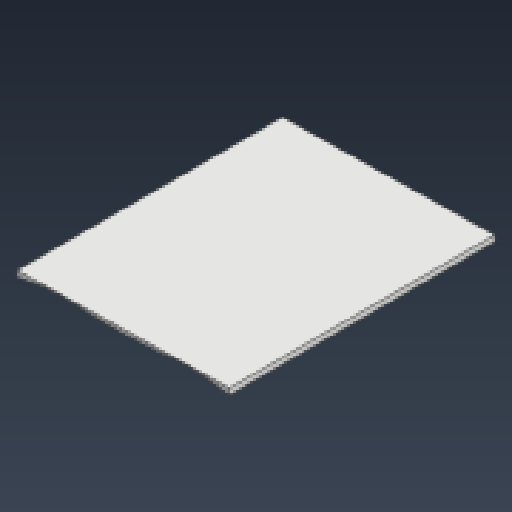
# Autodesk Inventor part: deseczka_dol_check - 6
Saved by Autodesk Inventor 2023 (Build 270158000, 158)
## iProperties
Created: 2025-12-25
Part Number: deseczka_dol_check - 6
Material: Generic
Document SubType Name: Modeling
Designer: szymo
Density: 1 g/cm^3
Appearance: Default
Author: szymo
Autodesk Inventor part; units mm, degrees
ref_plane "YZ Plane" through (0, 0, 0) normal (1, 0, 0) x (0, 1, 0)
ref_plane "XZ Plane" through (0, 0, 0) normal (0, 1, 0) x (-1, 0, 0)
sketch "Sketch1" plane through (0, 0, 0) normal (0, 0, 1) x (1, 0, 0)
  line L0 (0, 0) -> (293.4944, 0) construction
  line L1 (293.4944, 0) -> (293.4944, -132.0217) construction
  line L2 (293.4944, -132.0217) -> (0, -132.0217) construction
  line L3 (0, -132.0217) -> (0, 0) construction
  line L4 (79.3681, -56.3049) -> (159.3681, -56.3049) construction
  line L5 (283.1562, -93.1287) -> (274.2161, -88.6482) construction
  line L6 (283.1562, -93.1287) -> (282.3201, -93.1287) construction
  line L7 (18.3483, -97.5091) -> (27.4302, -93.3236) construction
  line L8 (18.3483, -97.5091) -> (20.5956, -97.5091) construction
  arc A0 (103.0994, -81.9859) -> (27.4302, -93.3236) centre (93.4367, -275.677) ccw
  arc A1 (274.2161, -88.6482) -> (204.4098, -79.893) centre (217.7822, -255.937) ccw
  arc A2 (103.0994, -81.9859) -> (204.4098, -79.893) centre (140.8276, 544.7964) ccw
  line L9 (27.4302, -93.3236) -> (27.4302, -72.2735)
  line L10 (27.4302, -72.2735) -> (272.6166, -67.591)
  line L11 (272.6166, -67.591) -> (274.2161, -88.6482)
  line L12 (103.0994, -81.9859) -> (86.3195, -71.1488) construction
  line L13 (204.4098, -79.893) -> (220.9707, -68.5773) construction
  line L14 (86.3195, -71.1488) -> (86.3195, -81.1488) construction
  line L15 (86.3195, -81.1488) -> (103.0994, -81.9859) construction
  line L16 (220.9707, -68.5773) -> (221.7303, -78.5773) construction
  line L17 (221.7303, -78.5773) -> (204.4098, -79.893) construction
  dimension "d5" = 80
  dimension "d85" = 10
  dimension "d87" = 26.619
  dimension "d92" = 10
  dimension "d94" = 24.743
  dimension "d100" = 22.985
  dimension "d101" = 22.755
  dimension "d106" = 10
  dimension "d111" = 10
  dimension "d112" = 30
  dimension "d113" = 30
  constraints: 28 end point, 6 point on circle, 5 horizontal, 3 centre point, 2 parallel, 2 point on line, 2 tangent, 1 perpendicular, 1 vertical, 8 other
  measures "d5" distance of L4.start L4.end
  measures "d85" distance of L5.start L5.end
  measures "d87" angle of L5 L6
  measures "d92" distance of L7.start L7.end
  measures "d94" angle of L7 L8
  measures "d106" distance of L12.end L14.end
  measures "d111" vertical distance of L13.end L16.end
  measures "d112" angle of L15 L12
  measures "d113" angle of L17 L13
extrude "Extrusion1" add sketch "Sketch1" along normal blind 10
sketch "Sketch2" plane through (0, 0, 10) normal (0, 0, 1) x (1, 0, 0)
  arc A0 (103.0994, -81.9859) -> (204.4098, -79.893) centre (140.8276, 544.7964) ccw projected
  line L0 (272.6166, -67.591) -> (27.4302, -72.2735) projected
  line L1 (27.4302, -72.2735) -> (27.4302, -93.3236) projected
  line L2 (274.2161, -88.6482) -> (272.6166, -67.591) projected
  line L3 (125.3768, -83.1204) -> (158.7723, -83.1204)
  line L4 (140.8276, -83.1204) -> (140.8276, -70.1078)
  line L5 (140.8276, -76.6141) -> (27.4302, -76.6141)
  line L6 (140.8276, -76.6141) -> (273.302, -76.6141)
  arc A1 (274.2161, -88.6482) -> (204.4098, -79.893) centre (217.7822, -255.937) ccw projected
  line L7 (274.2161, -88.6482) -> (272.6166, -67.591) projected
  line L8 (272.6166, -67.591) -> (27.4302, -72.2735) projected
  line L9 (27.4302, -72.2735) -> (27.4302, -93.3236) projected
  arc A2 (103.0994, -81.9859) -> (27.4302, -93.3236) centre (93.4367, -275.677) ccw projected
  arc A3 (103.0994, -81.9859) -> (204.4098, -79.893) centre (140.8276, 544.7964) ccw projected
  line L10 (140.8276, -83.1204) -> (140.4575, -63.7401)
  point P0 (0, 0)
  point P1 (204.4098, -79.893)
  point P2 (140.5792, -70.1126)
  point P3 (140.7034, -76.6141)
  dimension "d121" = 113.3974
  dimension "d122" = 132.4743
  constraints: 10 end point, 5 point on line, 3 horizontal, 2 perpendicular, 2 point on circle, 1 midpoint, 1 tangent
  measures "d121" distance of L5.start L5.end
  measures "d122" distance of L5.start L6.end
extrude "Extrusion2" cut sketch "Sketch2" against normal blind 10 contours L4 L6 L2 A1 A0 | L10 L5 L4 | L5 L10 L0 L4 | L4 L0 L2 L6
sketch "Sketch4" plane through (0, 0, 10) normal (0, 0, 1) x (1, 0, 0)
  line L0 (140.5792, -70.1126) -> (27.4302, -72.2735) projected
  line L1 (27.4302, -72.2735) -> (27.4302, -93.3236) projected
  arc A0 (103.0994, -81.9859) -> (27.4302, -93.3236) centre (93.4367, -275.677) ccw projected
  arc A1 (103.0994, -81.9859) -> (140.8276, -83.1204) centre (140.8276, 544.7964) ccw projected
  line L2 (27.4302, -72.2735) -> (27.4302, -93.3236) projected
  arc A2 (103.0994, -81.9859) -> (27.4302, -93.3236) centre (93.4367, -275.677) ccw projected
  line L3 (27.4302, -72.2735) -> (27.8295, -93.1796)
  line L4 (140.8276, -83.1204) -> (140.5792, -70.1126) projected
  point P0 (0, 0)
  point P1 (253.7282, -67.9517)
  dimension "d128" = 90
  constraints: 2 end point, 1 point on circle
  measures "d128" angle of L0 L3
extrude "Extrusion4" cut sketch "Sketch4" against normal blind 10 contours L3 A0 L1
sketch "Sketch6" plane through (0, 0, 10) normal (0, 0, 1) x (1, 0, 0)
  line L0 (27.4302, -72.2735) -> (27.8295, -93.1796) projected
  arc A0 (103.0994, -81.9859) -> (27.8295, -93.1796) centre (93.4367, -275.677) ccw projected
  arc A1 (103.0994, -81.9859) -> (140.8276, -83.1204) centre (140.8276, 544.7964) ccw projected
  line L1 (140.8276, -83.1204) -> (140.5792, -70.1126) projected
  line L2 (140.5792, -70.1126) -> (27.4302, -72.2735) projected
  line L3 (140.5792, -70.1126) -> (27.4302, -72.2735) projected
  line L4 (140.5792, -70.1126) -> (148.0778, -69.9694)
  line L5 (148.0778, -69.9694) -> (148.3263, -82.9772)
  line L6 (140.5792, -70.1126) -> (140.8276, -83.1204) projected
  line L7 (148.3263, -82.9772) -> (140.8276, -83.1204)
  point P0 (0, 0)
  dimension "d131" = 7.5
  dimension "d132" = 0
  dimension "d135" = 180
  constraints: 6 end point, 1 perpendicular
  measures "d131" distance of L1.end L4.end
  measures "d132" angle of L2 L7
  measures "d135" angle of L2 L4
extrude "Extrusion5" add sketch "Sketch6" against normal blind 10 contours L4 L5 L7 L1
sketch "Sketch7" plane through (0, 0, 10) normal (0, 0, 1) x (1, 0, 0)
  line L0 (27.4302, -72.2735) -> (27.8295, -93.1796) projected
  arc A0 (103.0994, -81.9859) -> (27.8295, -93.1796) centre (93.4367, -275.677) ccw projected
  arc A1 (103.0994, -81.9859) -> (140.8276, -83.1204) centre (140.8276, 544.7964) ccw projected
  line L1 (140.8276, -83.1204) -> (148.3263, -82.9772) projected
  line L2 (148.3263, -82.9772) -> (148.0778, -69.9694) projected
  line L3 (148.0778, -69.9694) -> (27.4302, -72.2735) projected
  line L4 (268.7255, -67.6653) -> (269.1247, -88.5714)
  arc A2 (269.1247, -88.5714) -> (193.4823, -80.2598) centre (210.5334, -273.4407) ccw
  arc A3 (155.8249, -82.834) -> (193.4823, -80.2598) centre (131.8501, 544.6249) ccw
  line L5 (155.8249, -82.834) -> (148.3263, -82.9772)
  line L6 (148.0778, -69.9694) -> (268.7255, -67.6653)
  point P0 (0, 0)
  constraints: 6 end point, 6 symmetric about line, 4 point on circle, 2 centre point, 2 other
extrude "Extrusion6" add sketch "Sketch7" against normal blind 10 contours L6 L4 A2 A3 L5 L2
sketch "Sketch8" plane through (0, 0, 10) normal (0, 0, 1) x (1, 0, 0)
  line L0 (27.4302, -72.2735) -> (27.8295, -93.1796) projected
  arc A0 (103.0994, -81.9859) -> (27.8295, -93.1796) centre (93.4367, -275.677) ccw projected
  arc A1 (103.0994, -81.9859) -> (140.8276, -83.1204) centre (140.8276, 544.7964) ccw projected
  line L1 (140.8276, -83.1204) -> (155.8249, -82.834) projected
  arc A2 (155.8249, -82.834) -> (193.4823, -80.2598) centre (131.8501, 544.6249) ccw projected
  arc A3 (269.1247, -88.5714) -> (193.4823, -80.2598) centre (210.5334, -273.4407) ccw projected
  line L2 (269.1247, -88.5714) -> (268.7255, -67.6653) projected
  line L3 (268.7255, -67.6653) -> (27.4302, -72.2735) projected
  line L4 (27.8295, -93.1796) -> (27.4302, -72.2735) projected
  line L5 (268.7255, -67.6653) -> (269.1247, -88.5714) projected
  line L6 (27.5859, -80.4275) -> (268.8812, -75.8193)
  point P0 (0, 0)
  dimension "d138" = 3
  constraints: 2 end point, 2 point on line, 1 parallel
  measures "d138" distance from line of A0.start L6
extrude "Extrusion7" cut sketch "Sketch8" against normal blind 10 contours L3 L2 L6 L0
sketch "Sketch9" plane through (0, 0, 0) normal (0, 0, -1) x (-1, 0, 0)
  line L0 (-27.5859, -80.4275) -> (-268.8812, -75.8193) projected
  line L1 (-268.8812, -75.8193) -> (-269.1247, -88.5714) projected
  arc A0 (-193.4823, -80.2598) -> (-269.1247, -88.5714) centre (-210.5334, -273.4407) ccw projected
  arc A1 (-193.4823, -80.2598) -> (-155.8249, -82.834) centre (-131.8501, 544.6249) ccw projected
  line L2 (-155.8249, -82.834) -> (-140.8276, -83.1204) projected
  arc A2 (-140.8276, -83.1204) -> (-103.0994, -81.9859) centre (-140.8276, 544.7964) ccw projected
  arc A3 (-27.8295, -93.1796) -> (-103.0994, -81.9859) centre (-93.4367, -275.677) ccw projected
  line L3 (-27.8295, -93.1796) -> (-27.5859, -80.4275) projected
  point P0 (0, 0)
extrude "Extrusion8" add sketch "Sketch9" along normal blind 10
sketch "Sketch10" plane through (0, 0, -10) normal (0, 0, -1) x (-1, 0, 0)
  line L0 (-27.5859, -80.4275) -> (-268.8812, -75.8193) projected
  line L1 (-268.8812, -75.8193) -> (-269.1247, -88.5714) projected
  arc A0 (-193.4823, -80.2598) -> (-269.1247, -88.5714) centre (-210.5334, -273.4407) ccw projected
  arc A1 (-193.4823, -80.2598) -> (-155.8249, -82.834) centre (-131.8501, 544.6249) ccw projected
  line L2 (-155.8249, -82.834) -> (-140.8276, -83.1204) projected
  arc A2 (-140.8276, -83.1204) -> (-103.0994, -81.9859) centre (-140.8276, 544.7964) ccw projected
  arc A3 (-27.8295, -93.1796) -> (-103.0994, -81.9859) centre (-93.4367, -275.677) ccw projected
  line L3 (-27.8295, -93.1796) -> (-27.5859, -80.4275) projected
  line L4 (-148.2336, -78.1234) -> (-148.3263, -82.9772)
  line L5 (-248.2153, -76.214) -> (-248.3494, -83.2315)
  line L6 (-48.3858, -87.0503) -> (-48.2518, -80.0328)
  line L7 (-268.8812, -75.8193) -> (-27.5859, -80.4275) projected
  point P0 (0, 0)
  dimension "d143" = 100
  dimension "d144" = 100
  constraints: 6 end point, 2 midpoint, 2 perpendicular, 2 point on circle, 2 point on line
  measures "d143" distance between parallel lines of L5 L4
  measures "d144" distance between parallel lines of L6 L4
extrude "Extrusion9" cut sketch "Sketch10" against normal through all contours L3 A3 L6 L0 | L5 A0 L1 L0
sketch "Sketch11" plane through (0, 0, 10) normal (0, 0, 1) x (1, 0, 0)
  line L0 (48.2518, -80.0328) -> (48.3858, -87.0503) projected
  arc A0 (103.0994, -81.9859) -> (48.3858, -87.0503) centre (93.4367, -275.677) ccw projected
  arc A1 (103.0994, -81.9859) -> (140.8276, -83.1204) centre (140.8276, 544.7964) ccw projected
  line L1 (140.8276, -83.1204) -> (155.8249, -82.834) projected
  arc A2 (155.8249, -82.834) -> (193.4823, -80.2598) centre (131.8501, 544.6249) ccw projected
  arc A3 (248.3494, -83.2315) -> (193.4823, -80.2598) centre (210.5334, -273.4407) ccw projected
  line L2 (248.3494, -83.2315) -> (248.2153, -76.214) projected
  line L3 (248.2153, -76.214) -> (48.2518, -80.0328) projected
  line L4 (48.2812, -81.5719) -> (248.2447, -77.753)
  circle A4 centre (93.4367, -275.677) radius 194.9319
  circle A5 centre (210.5334, -273.4407) radius 194.9319
  point P0 (0, 0)
  dimension "d147" = 1
  dimension "d148" = 1
  constraints: 2 centre point, 2 coincident, 2 end point, 2 point on line, 2 tangent, 1 parallel, 1 perpendicular
  measures "d147" radial gap between concentric circles of A4 A0
  measures "d148" radial gap between concentric circles of A3 A5
extrude "Extrusion10" cut sketch "Sketch11" against normal through all contours L3 L2 L4 L0
sketch "Sketch12" plane through (0, 0, 10) normal (0, 0, 1) x (1, 0, 0)
  line L0 (248.2447, -77.753) -> (48.2812, -81.5719) projected
  line L1 (48.2812, -81.5719) -> (48.3858, -87.0503) projected
  arc A0 (103.0994, -81.9859) -> (48.3858, -87.0503) centre (93.4367, -275.677) ccw projected
  arc A1 (103.0994, -81.9859) -> (140.8276, -83.1204) centre (140.8276, 544.7964) ccw projected
  line L2 (140.8276, -83.1204) -> (155.8249, -82.834) projected
  arc A2 (155.8249, -82.834) -> (193.4823, -80.2598) centre (131.8501, 544.6249) ccw projected
  arc A3 (248.3494, -83.2315) -> (193.4823, -80.2598) centre (210.5334, -273.4407) ccw projected
  line L3 (248.3494, -83.2315) -> (248.2447, -77.753) projected
  point P0 (0, 0)
ref_plane "Work Plane2" through (47.6702, -81.5719, 240) normal (0, 0, -1) x (-0.0191, 0.9998, 0)
extrude "Extrusion11" add sketch "Sketch12" along normal up to surface (230 mm away)
equation "\"d111\" = d106"
equation "\"d113\" = d112"
body "Solid1"
